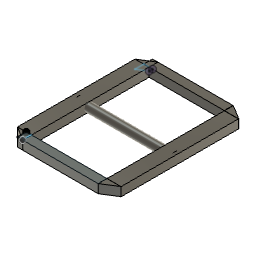
3d_4 (Autodesk Fusion 360 design; units mm, degrees)
Autodesk Fusion 360 part; units mm, degrees
cylinder "CylinderPrimitive1" add diameter 5 height 55 placed x (1, 0, 0) y (0, 1, 0) z (0, 0, 1) at (0, 0, 0) makes body 1
move_body "Move1" bodies 1 to x (0, 0, -1) y (0, 1, 0) z (1, 0, 0) at (-5, 0, -5)
move_body "Move2" bodies 1 to x (1, 0, 0) y (0, 1, 0) z (0, 0, 1) at (0, 0, 10)
box "BoxPrimitive1" add length 67 width 8 height 5 placed x (0, -1, 0) y (1, 0, 0) z (0, 0, 1) at (65, 30, 0) separate body makes body 2
move_body "Move4" bodies 2 to x (1, 0, 0) y (0, 1, 0) z (0, 0, 1) at (-21, 0, 0)
move_face "MoveFace1" to x (1, 0, 0) y (0, 1, 0) z (0, 0, 1) at (0, 4.5389, -2.0973) 1 faces at (31.6667, -0.2489, 2.5124) on bodies 1
move_face "MoveFace2" to x (1, 0, 0) y (0, 1, 0) z (0, 0, 1) at (0, 0.8539, -0.5205) 1 faces at (31.6667, 4.2899, 0.4151) on bodies 1
move_face "MoveFace3" to x (1, 0, 0) y (0, 1, 0) z (0, 0, 1) at (0, -4.9281, -0.8448) 1 faces at (31.6667, 5.1438, -0.1054) on bodies 1
move_face "MoveFace4" to x (1, 0, 0) y (0, 1, 0) z (0, 0, 1) at (0, -0.9976, 0.0687) 1 faces at (31.6667, 0.2157, -0.9502) on bodies 1
move_face "MoveFace5" to x (1, 0, 0) y (0, 1, 0) z (0, 0, 1) at (0, 0.4635, 0.1875) 1 faces at (31.6667, -0.782, -0.8815) on bodies 1
move_face "MoveFace6" to x (1, 0, 0) y (0, 1, 0) z (0, 0, 1) at (0.5, 0, 0) 1 faces at (31.6667, -0.3185, -0.694) on bodies 1
move_face "MoveFace7" to x (1, 0, 0) y (0, 1, 0) z (0, 0, 1) at (0, -0.0778, 0.4939) 1 faces at (31.6667, -0.3185, -0.694) on bodies 1
move_face "MoveFace8" to x (1, 0, 0) y (0, 1, 0) z (0, 0, 1) at (0, 0.2336, 0.4421) 1 faces at (31.6667, -0.3962, -0.2001) on bodies 1
move_face "MoveFace9" to x (1, 0, 0) y (0, 1, 0) z (0, 0, 1) at (0, 0.0954, -0.2844) 1 faces at (31.6667, -0.1627, 0.242) on bodies 1
move_body "Move6" bodies 2 to x (1, 0, 0) y (0, 1, 0) z (0, 0, 1) at (0, 4.5, 0)
copy_body "CopyPasteBodies2" bodies 2 makes body 3
move_body "Move7" bodies 3 to x (1, 0, 0) y (0, 1, 0) z (0, 0, 1) at (-48, 0, 0)
move_body "Move8" bodies 3 to x (1, 0, 0) y (0, 1, 0) z (0, 0, 1) at (-2, 0, 0)
move_body "Move9" bodies 3 to x (1, 0, 0) y (0, 1, 0) z (0, 0, 1) at (-1, 0, 0)
move_body "Move10" bodies 3 to x (1, 0, 0) y (0, 1, 0) z (0, 0, 1) at (-3, 0, 0)
sketch "Sketch9" plane through (0, 0, 0) normal (0, 1, 0) x (1, 0, 0)
  line L0 (44, -5, 34.5) -> (-2, -5, 34.5)
  line L1 (-2, -5, 34.5) -> (-2, 0, 34.5)
  line L2 (-2, 0, 34.5) -> (44, 0, 34.5)
  line L3 (44, 0, 34.5) -> (44, -5, 34.5)
extrude "Extrude1" add sketch "Sketch9" along normal blind 5 separate body contours L0 L1 L2 L3 in plane through (0, 34.5, 0) normal (0, 1, 0) makes body 4
sketch "Sketch10" plane through (0, 0, 0) normal (0, 1, 0) x (1, 0, 0)
sketch "Sketch11" plane through (0, 0, 0) normal (0, 0, 1) x (1, 0, 0)
sketch "Sketch12" plane through (0, 0, 0) normal (0, 0, 1) x (1, 0, 0)
  line L0 (43.8263, 39.4632) -> (52.0112, 39.4632)
  line L1 (52.0112, 34.6148) -> (52.0112, 34.3947)
  line L2 (52.0112, 34.3947) -> (43.8263, 34.3947)
  line L3 (43.8263, 34.3947) -> (43.8263, 39.4632)
  line L4 (44.0478, 39.4632) -> (52.0112, 34.6148)
  constraint horizontal L0
  constraint vertical L1
  constraint horizontal L2
  constraint vertical L3
  constraint coincident L0 L4.start
extrude "Extrude2" add sketch "Sketch12" along normal blind 5 separate body makes body 5
sketch "Sketch13" plane through (0, 0, 0) normal (0, 0, 1) x (1, 0, 0)
  line L0 (-1.9573, 34.4559) -> (-9.9871, 34.4559)
  line L1 (-1.9573, 39.4935) -> (-1.9573, 34.4559)
  line L2 (-1.9573, 39.4935) -> (-9.9871, 34.4559)
  constraint horizontal L0
  constraint vertical L1
extrude "Extrude3" add sketch "Sketch13" along normal blind 5 separate body makes body 6
sketch "Sketch14" plane through (0, 0, 0) normal (1, 0, 0) x (0, 1, 0)
sketch "Sketch15" plane through (0, 0, 0) normal (0, 1, 0) x (1, 0, 0)
  line L0 (-2, -5, -32.5) -> (44, -5, -32.5)
  line L1 (44, -5, -32.5) -> (44, 0, -32.5)
  line L2 (44, 0, -32.5) -> (-2, 0, -32.5)
  line L3 (-2, 0, -32.5) -> (-2, -5, -32.5)
  point P0 (-2, -5)
  point P1 (44, 0)
extrude "Extrude4" add sketch "Sketch15" along normal blind 5 separate body contours L0 L1 L2 L3 in plane through (0, -32.5, 0) normal (0, 1, 0) makes body 7
move_body "Move11" bodies 7 to x (1, 0, 0) y (0, 1, 0) z (0, 0, 1) at (0, -5, 0)
copy_body "CopyPasteBodies3" bodies 6 makes body 8
move_body "Move12" bodies 8 to x (1, 0, 0) y (0, 1, 0) z (0, 0, 1) at (0, -70, 0)
move_body "Move13" bodies 8 to x (-1, 0, 0) y (0, -1, 0) z (0, 0, 1) at (-3.9145, -71.0883, 0)
move_body "Move14" bodies 8 to x (1, 0, 0) y (0, 1, 0) z (0, 0, 1) at (46, 3, 0)
move_body "Move15" bodies 8 to x (1, 0, 0) y (0, 1, 0) z (0, 0, 1) at (-0.1, 0.1, 0)
move_body "Move16" bodies 6 to x (1, 0, 0) y (0, 1, 0) z (0, 0, 1) at (0, -70, 0)
move_body "Move17" bodies 6 to x (0, -1, 0) y (1, 0, 0) z (0, 0, 1) at (25.557, -45.5313, 0)
move_body "Move18" bodies 6 to x (-0.435154, -0.900356, 0) y (-0.900356, 0.435154, 0) z (0, 0, -1) at (-46.3354, -29.0689, 10)
move_body "Move19" bodies 6 to x (1, 0, 0) y (0, 1, 0) z (0, 0, 1) at (0, 0, -5)
move_body "Move20" bodies 6 to x (0.906308, 0.422618, 0) y (-0.422618, 0.906308, 0) z (0, 0, 1) at (-16.7567, -2.4923, 0)
move_body "Move21" bodies 6 to x (1, 0, 0) y (0, 1, 0) z (0, 0, 1) at (0, 6, 0)
move_body "Move22" bodies 6 to x (0.999848, 0.017452, 0) y (-0.017452, 0.999848, 0) z (0, 0, 1) at (-0.6649, 0.0435, 0)
move_body "Move23" bodies 6 to x (1, 0, 0) y (0, 1, 0) z (0, 0, 1) at (0.95, 0.51, 0)
sketch "Sketch16" plane through (0, 0, 0) normal (0, 0, 1) x (1, 0, 0)
  line L0 (-1.9357, 34.4298) -> (-9.9675, 34.4298)
  line L1 (-1.9357, 39.521) -> (-1.9357, 34.4298)
  line L2 (-1.9357, 39.521) -> (-9.9675, 34.4298)
  constraint horizontal L0
  constraint vertical L1
extrude "Extrude5" add sketch "Sketch16" along normal blind 5 separate body makes body 9
move_body "Move24" bodies 3 to x (1, 0, 0) y (0, 1, 0) z (0, 0, 1) at (3, 0, 0)
move_body "Move25" bodies 9 to x (1, 0, 0) y (0, 1, 0) z (0, 0, 1) at (3, 0, 0)
sketch "Sketch17" plane through (0, 0, 0) normal (0, 0, 1) x (1, 0, 0)
  line L0 (-2.1495, 39.5134) -> (-7, 39.5134)
  line L1 (-7, 39.5134) -> (-7, 34.5134)
  line L2 (-7, 34.5134) -> (-2, 37.5134)
  constraint horizontal L0
  constraint perpendicular L0 L1
sketch "Sketch18" plane through (0, 0, 0) normal (0, 0, 1) x (1, 0, 0)
  line L0 (-2, 39.5) -> (-2, 37.5134)
  point P0 (-2, 39.5)
  point P1 (-2, 37.5134)
  constraint coincident P0 L0.start
  constraint coincident P1 L0.end
sketch "Sketch19" plane through (0, 0, 5) normal (0, 0, 1) x (-1, 0, 0)
  line L0 (2, 37.5) -> (-44, 37.5)
  line L1 (-44, 37.5) -> (-44, 32.5)
  line L2 (-44, 32.5) -> (2, 32.5)
  line L3 (2, 32.5) -> (2, 37.5)
  line L4 (2, 32.5) -> (-0.9653, 32.5)
  line L5 (-0.9653, 32.5) -> (-0.9653, 37.5)
  line L6 (-0.9653, 37.5) -> (2, 37.5)
  line L7 (2, 37.5) -> (2, 32.5)
  constraint horizontal L4
  constraint vertical L5
  constraint horizontal L6
  constraint vertical L7
  constraint coincident L0 L5.end
  constraint coincident L2.end L3.start
move_body "Move26" bodies 6 to x (1, 0, 0) y (0, 1, 0) z (0, 0, 1) at (3, 0, 0)
